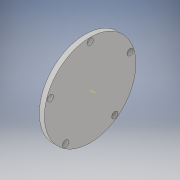
# Autodesk Inventor part: lip plate
Saved by Autodesk Inventor 2018 (Build 220112000, 112)
## iProperties
Created: 2021-03-15
Part Number: lip plate
Material: Generic
Document SubType Name: Modeling
Designer: Jyoti Soni
Density: 1 g/cm^3
Appearance: Default
Author: Jyoti Soni
Autodesk Inventor part; units mm, degrees
ref_plane "YZ Plane" through (0, 0, 0) normal (1, 0, 0) x (0, 1, 0)
ref_plane "XZ Plane" through (0, 0, 0) normal (0, 1, 0) x (-1, 0, 0)
ref_plane "XY Plane" through (0, 0, 0) normal (0, 0, 1) x (1, 0, 0)
sketch "Sketch1" plane through (0, 0, 0) normal (1, 0, 0) x (0, 1, 0)
  circle A0 centre (0, 0) radius 90
  dimension "d0" = 180
  constraints: 1 centre point, 1 coincident
  measures "d0" diameter of A0
extrude "Extrusion1" add sketch "Sketch1" along normal blind 10
sketch "Sketch2" plane through (10, 0, 0) normal (1, 0, 0) x (0, 0, -1)
  circle A0 centre (0, 82.5) radius 6
  point P0 (0, 0)
  dimension "d3" = 82.5
  dimension "d4" = 12
  constraints: 1 centre point
  measures "d3" distance of A0.centre point (0, 0)
  measures "d4" diameter of A0
extrude "Extrusion2" cut sketch "Sketch2" against normal blind 10
pattern_circular "Circular Pattern1" count 5 over 360 about axis through (10, 0, 0) along (1, 0, 0) of "Extrusion2"
body "Solid1"
